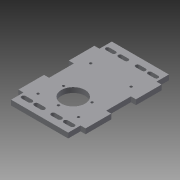
# Autodesk Inventor part: bottom
Saved by Autodesk Inventor 2015 (Build 190159000, 159)
## iProperties
Created: 2017-03-04
Part Number: bottom
Material: Generic
Document SubType Name: Modeling
Designer: Guy
Density: 1 g/cm^3
Appearance: Default
Author: Guy
Autodesk Inventor part; units mm, degrees
ref_plane "YZ Plane" through (0, 0, 0) normal (1, 0, 0) x (0, 1, 0)
ref_plane "XZ Plane" through (0, 0, 0) normal (0, 1, 0) x (-1, 0, 0)
ref_plane "XY Plane" through (0, 0, 0) normal (0, 0, 1) x (1, 0, 0)
sketch "Sketch1" plane through (0, 0, 0) normal (0, 0, 1) x (1, 0, 0)
  line L0 (0, 0) -> (120, 0)
  line L1 (120, 0) -> (120, 80)
  line L2 (120, 80) -> (0, 80)
  line L3 (0, 80) -> (0, 0)
  dimension "d0" = 120
  dimension "d1" = 80
  constraints: 8 end point, 2 parallel, 1 horizontal, 1 perpendicular
  measures "d0" distance of L2.end L1.end
  measures "d1" distance of L0.end L1.end
extrude "Extrusion1" add sketch "Sketch1" along normal blind 6
sketch "Sketch2" plane through (0, 0, 6) normal (0, 0, 1) x (1, 0, 0)
  line L0 (0, 0) -> (120, 0) projected
  line L1 (120, 0) -> (120, 80) projected
  line L2 (120, 80) -> (0, 80) projected
  line L3 (0, 80) -> (0, 0) projected
  line L4 (120, 0) -> (105.25, 0)
  line L5 (105.25, 0) -> (105.25, 6)
  line L6 (105.25, 6) -> (120, 6)
  line L7 (120, 6) -> (120, 0)
  line L8 (0, 0) -> (120, 0) projected
  line L9 (74.75, 0) -> (45.25, 0)
  line L10 (45.25, 0) -> (45.25, 6)
  line L11 (45.25, 6) -> (74.75, 6)
  line L12 (74.75, 6) -> (74.75, 0)
  line L13 (14.75, 0) -> (0, 0)
  line L14 (0, 0) -> (0, 6)
  line L15 (0, 6) -> (14.75, 6)
  line L16 (14.75, 6) -> (14.75, 0)
  line L17 (120, 80) -> (105.25, 80)
  line L18 (105.25, 80) -> (105.25, 74)
  line L19 (105.25, 74) -> (120, 74)
  line L20 (120, 74) -> (120, 80)
  line L21 (120, 80) -> (0, 80) projected
  line L22 (74.75, 80) -> (45.25, 80)
  line L23 (45.25, 80) -> (45.25, 74)
  line L24 (45.25, 74) -> (74.75, 74)
  line L25 (74.75, 74) -> (74.75, 80)
  line L26 (14.75, 80) -> (0, 80)
  line L27 (0, 80) -> (0, 74)
  line L28 (0, 74) -> (14.75, 74)
  line L29 (14.75, 74) -> (14.75, 80)
  line L30 (60, -24.5918) -> (60, 107.6161)
  line L31 (0, 80) -> (0, 0) projected
  dimension "d4" = 6
  dimension "d5" = 6
  dimension "d6" = 14.75
  dimension "d7" = 14.75
  dimension "d8" = 29.5
  dimension "d18" = 60
  dimension "d19" = 14.75
  constraints: 50 end point, 13 parallel, 10 point on line, 6 horizontal, 6 perpendicular, 4 collinear
  measures "d4" distance between parallel lines of L6 L4
  measures "d5" distance between parallel lines of L26 L28
  measures "d6" distance between parallel lines of L5 L1
  measures "d7" distance between parallel lines of L16 L14
  measures "d8" distance between parallel lines of L12 L10
  measures "d18" distance between parallel lines of L3 L30
  measures "d19" distance between parallel lines of L12 L30
extrude "Extrusion2" cut sketch "Sketch2" against normal up to next contours L3 L15 L16 L0 | L10 L11 L30 L0 | L3 L2 L29 L28 | L30 L11 L12 L0 | L5 L6 L1 L0 | L30 L2 L25 L24 | L24 L23 L2 L30 | L19 L18 L2 L1
sketch "Sketch3" plane through (0, 0, 6) normal (0, 0, 1) x (1, 0, 0)
  circle A0 centre (80, 40) radius 4.6
  line L0 (74.75, 0) -> (105.25, 0) projected
  line L1 (120, 6) -> (120, 74) projected
  point P0 (0, 0)
  dimension "d13" = 9.2
  dimension "d14" = 40
  dimension "d15" = 40
  constraints: 1 centre point
  measures "d13" diameter of A0
  measures "d14" distance from line of A0.centre L0
  measures "d15" distance from line of L1 A0.centre
extrude "Extrusion3" cut sketch "Sketch3" against normal up to next
sketch "Sketch4" plane through (0, 0, 6) normal (0, 0, 1) x (1, 0, 0)
  circle A0 centre (80, 40) radius 4.6 projected
  line L0 (74.75, 6) -> (74.75, 0) projected
  line L1 (74.75, 0) -> (105.25, 0) projected
  line L2 (105.25, 0) -> (105.25, 6) projected
  line L3 (105.25, 6) -> (120, 6) projected
  line L4 (120, 6) -> (120, 74) projected
  line L5 (120, 74) -> (105.25, 74) projected
  line L6 (105.25, 74) -> (105.25, 80) projected
  line L7 (105.25, 80) -> (74.75, 80) projected
  line L8 (74.75, 80) -> (74.75, 74) projected
  line L9 (74.75, 74) -> (45.25, 74) projected
  line L10 (45.25, 74) -> (45.25, 80) projected
  line L11 (45.25, 80) -> (14.75, 80) projected
  line L12 (14.75, 80) -> (14.75, 74) projected
  line L13 (14.75, 74) -> (0, 74) projected
  line L14 (0, 74) -> (0, 6) projected
  line L15 (0, 6) -> (14.75, 6) projected
  line L16 (14.75, 6) -> (14.75, 0) projected
  line L17 (14.75, 0) -> (45.25, 0) projected
  line L18 (45.25, 0) -> (45.25, 6) projected
  line L19 (45.25, 6) -> (74.75, 6) projected
  circle A1 centre (80, 40) radius 14.125
  circle A2 centre (97.5, 40) radius 1.5
  circle A3 centre (74.5, 57) radius 1.5
  circle A4 centre (74.5, 23) radius 1.5
  circle A5 centre (35.064, 64.1) radius 1.5
  circle A6 centre (35.064, 15.9) radius 1.5
  line L20 (80, 40) -> (97.5, 40) construction
  circle A7 centre (10, 66.125) radius 2.3
  circle A8 centre (10, 51.125) radius 2.3
  circle A9 centre (10, 13.875) radius 2.3
  circle A10 centre (10, 28.875) radius 2.3
  circle A11 centre (110, 66.125) radius 2.5
  circle A12 centre (110, 51.125) radius 2.5
  circle A13 centre (110, 13.875) radius 2.5
  circle A14 centre (110, 28.875) radius 2.5
  line L21 (10, 66.125) -> (110, 66.125) construction
  line L22 (110, 66.125) -> (110, 13.875) construction
  line L23 (110, 13.875) -> (10, 13.875) construction
  line L24 (10, 13.875) -> (10, 66.125) construction
  circle A15 centre (10, 61.125) radius 2.3
  circle A16 centre (10, 54.125) radius 2.3
  circle A17 centre (10, 69.125) radius 2.3
  circle A18 centre (10, 46.525) radius 2.3
  circle A19 centre (10, 33.475) radius 2.3
  circle A20 centre (10, 25.875) radius 2.3
  circle A21 centre (10, 18.475) radius 2.3
  circle A22 centre (10, 10.875) radius 2.3
  circle A23 centre (110, 69.125) radius 2.5
  circle A24 centre (110, 61.125) radius 2.5
  circle A25 centre (110, 54.125) radius 2.5
  circle A26 centre (110, 46.125) radius 2.5
  circle A27 centre (110, 33.875) radius 2.5
  circle A28 centre (110, 25.875) radius 2.5
  circle A29 centre (110, 18.875) radius 2.5
  circle A30 centre (110, 10.875) radius 2.5
  line L25 (7.7, 69.125) -> (7.7, 61.125)
  line L26 (12.3, 61.125) -> (12.3, 69.125)
  line L27 (7.7, 54.125) -> (7.7, 46.525)
  line L28 (12.3, 46.525) -> (12.3, 54.125)
  line L29 (7.7, 10.875) -> (7.7, 18.475)
  line L30 (7.7, 25.875) -> (7.7, 33.475)
  line L31 (12.3, 33.475) -> (12.3, 25.875)
  line L32 (12.3, 18.475) -> (12.3, 10.875)
  line L33 (112.5, 61.125) -> (112.5, 69.125)
  line L34 (107.5, 69.125) -> (107.5, 61.125)
  line L35 (107.5, 54.125) -> (107.5, 46.125)
  line L36 (112.5, 46.125) -> (112.5, 54.125)
  line L37 (107.5, 33.875) -> (107.5, 25.875)
  line L38 (107.5, 18.875) -> (107.5, 10.875)
  line L39 (112.5, 10.875) -> (112.5, 18.875)
  line L40 (112.5, 25.875) -> (112.5, 33.875)
  point P0 (0, 0)
  dimension "d20" = 28.25
  dimension "d21" = 3
  dimension "d22" = 3
  dimension "d23" = 3
  dimension "d24" = 3
  dimension "d25" = 3
  dimension "d26" = 17.5
  dimension "d27" = 5.5
  dimension "d28" = 5.5
  dimension "d29" = 34
  dimension "d30" = 17
  dimension "d31" = 48.2
  dimension "d32" = 24.1
  dimension "d33" = 44.936
  dimension "d34" = 44.936
  dimension "d37" = 10
  dimension "d38" = 10
  dimension "d39" = 4.6
  dimension "d40" = 4.6
  dimension "d41" = 4.6
  dimension "d42" = 4.6
  dimension "d43" = 5
  dimension "d44" = 5
  dimension "d45" = 5
  dimension "d46" = 5
  dimension "d47" = 13.875
  dimension "d48" = 13.875
  dimension "d49" = 15
  dimension "d50" = 15
  dimension "d51" = 15
  dimension "d52" = 15
  dimension "d53" = 4.6
  dimension "d54" = 4.6
  dimension "d56" = 3
  dimension "d57" = 5
  dimension "d58" = 4.6
  dimension "d59" = 3
  dimension "d60" = 4.6
  dimension "d61" = 4.6
  dimension "d62" = 4.6
  dimension "d63" = 4.6
  dimension "d64" = 4.6
  dimension "d65" = 3
  dimension "d66" = 3
  dimension "d67" = 5
  dimension "d68" = 5
  dimension "d69" = 5
  dimension "d70" = 5
  dimension "d71" = 5
  dimension "d72" = 5
  dimension "d73" = 5
  dimension "d74" = 5
  dimension "d75" = 3
  dimension "d76" = 3
  dimension "d77" = 3
  dimension "d78" = 3
  constraints: 38 end point, 34 tangent, 32 point on circle, 30 centre point, 4 vertical, 3 coincident, 3 horizontal, 1 parallel, 1 point on line, 26 other
  measures "d20" diameter of A1
  measures "d21" diameter of A5
  measures "d22" diameter of A6
  measures "d23" diameter of A3
  measures "d24" diameter of A4
  measures "d25" diameter of A2
  measures "d26" distance of A0.centre L20.end
  measures "d27" horizontal distance of A0.centre A3.centre
  measures "d28" horizontal distance of A0.centre A4.centre
  measures "d29" distance of A3.centre A4.centre
  measures "d30" vertical distance of A3.centre L20.start
  measures "d31" distance of A6.centre A5.centre
  measures "d32" vertical distance of A0.centre A5.centre
  measures "d33" horizontal distance of A0.centre A5.centre
  measures "d34" horizontal distance of L20.start A6.centre
  measures "d39" diameter of A7
  measures "d40" diameter of A8
  measures "d41" diameter of A9
  measures "d42" diameter of A10
  measures "d43" diameter of A13
  measures "d44" diameter of A14
  measures "d45" diameter of A12
  measures "d46" diameter of A11
  measures "d47" distance between parallel lines of L11 L21
  measures "d48" distance between parallel lines of L23 L17
  measures "d49" distance of A8.centre L21.start
  measures "d50" distance of A9.centre A10.centre
  measures "d51" distance of A12.centre A11.centre
  measures "d52" distance from line of L23 A14.centre
  measures "d53" diameter of A15
  measures "d54" diameter of A16
  measures "d56" distance of A16.centre A8.centre
  measures "d57" distance of A15.centre L21.start
  measures "d58" diameter of A17
  measures "d59" distance of L21.start A17.centre
  measures "d60" diameter of A18
  measures "d61" diameter of A19
  measures "d62" diameter of A20
  measures "d63" diameter of A21
  measures "d64" diameter of A22
  measures "d65" distance of A9.centre A22.centre
  measures "d66" distance of A10.centre A20.centre
  measures "d67" diameter of A23
  measures "d68" diameter of A24
  measures "d69" diameter of A25
  measures "d70" diameter of A26
  measures "d71" diameter of A27
  measures "d72" diameter of A28
  measures "d73" diameter of A29
  measures "d74" diameter of A30
  measures "d75" distance of L23.start A30.centre
  measures "d76" distance of A11.centre A23.centre
  measures "d77" distance of A12.centre A25.centre
  measures "d78" distance of A14.centre A28.centre
extrude "Extrusion4" cut sketch "Sketch4" against normal blind 10 contours A1 | A2 | A3 | A4 | A5 | A6
extrude "Extrusion5" cut sketch "Sketch4" against normal blind 10 contours A7 A17 | L26 A15 L25 A7 | A7 A17 L26 | A17 A7 | A7 A17 | L25 A17 A7 | A15 | A8 A16 | L28 A18 A8 | A8 A16 L28 | A16 A8 | A8 A16 | A18 L27 A8 | A18 | A8 L27 A16 | A9 A22 | L32 A22 A9 | A9 A21 L32 | A9 L29 A21 | A21 | A22 A9 | A9 A22 | A9 A22 L29 | A10 A20 | L31 A20 A10 | A10 A19 L31 | A10 L30 A19 | A19 | A20 A10 | A10 A20 | A10 A20 L30 | A11 A23 | L33 A24 A11 | A11 A23 L33 | A23 A11 | A11 A23 | A24 L34 A11 | A24 | A11 L34 A23 | A12 A25 | L36 A26 A12 | A12 A25 L36 | A25 A12 | A12 A25 | A26 L35 A12 | A26 | A12 L35 A25 | A13 A30 | L39 A30 A13 | A13 A29 L39 | A13 L38 A29 | A29 | A30 A13 | A13 A30 | A13 A30 L38 | A14 A28 | L40 A28 A14 | A14 A27 L40 | A14 L37 A27 | A27 | A28 A14 | A14 A28 | A14 A28 L37
sketch "Sketch6" plane through (0, 0, 6) normal (0, 0, 1) x (1, 0, 0)
  line L0 (107.5, 25.875) -> (107.5, 33.875) projected
  arc A0 (112.5, 33.875) -> (107.5, 33.875) centre (110, 33.875) ccw projected
  line L1 (112.5, 33.875) -> (112.5, 25.875) projected
  arc A1 (107.5, 25.875) -> (112.5, 25.875) centre (110, 25.875) ccw projected
  line L2 (7.7, 25.875) -> (7.7, 33.475) projected
  arc A2 (12.3, 33.475) -> (7.7, 33.475) centre (10, 33.475) ccw projected
  line L3 (12.3, 33.475) -> (12.3, 25.875) projected
  arc A3 (7.7, 25.875) -> (12.3, 25.875) centre (10, 25.875) ccw projected
  line L4 (12.3, 54.125) -> (12.3, 46.525) projected
  arc A4 (7.7, 46.525) -> (12.3, 46.525) centre (10, 46.525) ccw projected
  line L5 (7.7, 46.525) -> (7.7, 54.125) projected
  arc A5 (12.3, 54.125) -> (7.7, 54.125) centre (10, 54.125) ccw projected
  line L6 (7.7, 10.875) -> (7.7, 18.475) projected
  arc A6 (12.3, 18.475) -> (7.7, 18.475) centre (10, 18.475) ccw projected
  line L7 (12.3, 18.475) -> (12.3, 10.875) projected
  arc A7 (7.7, 10.875) -> (12.3, 10.875) centre (10, 10.875) ccw projected
  line L8 (107.5, 61.125) -> (107.5, 69.125) projected
  arc A8 (112.5, 69.125) -> (107.5, 69.125) centre (110, 69.125) ccw projected
  line L9 (112.5, 69.125) -> (112.5, 61.125) projected
  arc A9 (107.5, 61.125) -> (112.5, 61.125) centre (110, 61.125) ccw projected
  line L10 (112.5, 18.875) -> (112.5, 10.875) projected
  arc A10 (107.5, 10.875) -> (112.5, 10.875) centre (110, 10.875) ccw projected
  line L11 (107.5, 10.875) -> (107.5, 18.875) projected
  arc A11 (112.5, 18.875) -> (107.5, 18.875) centre (110, 18.875) ccw projected
  line L12 (7.7, 61.125) -> (7.7, 69.125) projected
  arc A12 (12.3, 69.125) -> (7.7, 69.125) centre (10, 69.125) ccw projected
  line L13 (12.3, 69.125) -> (12.3, 61.125) projected
  arc A13 (7.7, 61.125) -> (12.3, 61.125) centre (10, 61.125) ccw projected
  line L14 (112.5, 54.125) -> (112.5, 46.125) projected
  arc A14 (107.5, 46.125) -> (112.5, 46.125) centre (110, 46.125) ccw projected
  line L15 (107.5, 46.125) -> (107.5, 54.125) projected
  arc A15 (112.5, 54.125) -> (107.5, 54.125) centre (110, 54.125) ccw projected
  circle A16 centre (80, 40) radius 14.125 projected
  circle A17 centre (35.064, 64.1) radius 1.5 projected
  circle A18 centre (74.5, 57) radius 1.5 projected
  circle A19 centre (97.5, 40) radius 1.5 projected
  circle A20 centre (74.5, 23) radius 1.5 projected
  circle A21 centre (35.064, 15.9) radius 1.5 projected
  line L16 (74.75, 6) -> (74.75, 0) projected
  line L17 (74.75, 0) -> (105.25, 0) projected
  line L18 (105.25, 0) -> (105.25, 6) projected
  line L19 (105.25, 6) -> (120, 6) projected
  line L20 (120, 6) -> (120, 74) projected
  line L21 (120, 74) -> (105.25, 74) projected
  line L22 (105.25, 74) -> (105.25, 80) projected
  line L23 (105.25, 80) -> (74.75, 80) projected
  line L24 (74.75, 80) -> (74.75, 74) projected
  line L25 (74.75, 74) -> (45.25, 74) projected
  line L26 (45.25, 74) -> (45.25, 80) projected
  line L27 (45.25, 80) -> (14.75, 80) projected
  line L28 (14.75, 80) -> (14.75, 74) projected
  line L29 (14.75, 74) -> (0, 74) projected
  line L30 (0, 74) -> (0, 6) projected
  line L31 (0, 6) -> (14.75, 6) projected
  line L32 (14.75, 6) -> (14.75, 0) projected
  line L33 (14.75, 0) -> (45.25, 0) projected
  line L34 (45.25, 0) -> (45.25, 6) projected
  line L35 (45.25, 6) -> (74.75, 6) projected
  circle A22 centre (97.765, 15.9) radius 1.5
  circle A23 centre (97.765, 64.1) radius 1.5
  point P0 (0, 0)
  dimension "d94" = 62.701
  dimension "d95" = 15.9
  dimension "d96" = 15.9
  dimension "d97" = 3
  dimension "d98" = 62.701
  dimension "d99" = 15.9
  dimension "d100" = 3
  constraints: 2 centre point
  measures "d94" distance of A22.centre A21.centre
  measures "d95" distance from line of L33 A21.centre
  measures "d96" distance from line of L17 A22.centre
  measures "d97" diameter of A22
  measures "d98" distance of A17.centre A23.centre
  measures "d99" distance from line of L23 A23.centre
  measures "d100" diameter of A23
extrude "Extrusion7" cut sketch "Sketch6" against normal blind 10 contours A22 | A23
equation "\"d22\" = d21"
equation "\"d23\" = d21"
equation "\"d24\" = d21"
equation "\"d25\" = d21"
equation "\"d30\" = 0.5 * d29"
equation "\"d32\" = 0.5 * d31"
equation "\"d34\" = d33"
equation "\"d39\" = d64"
equation "\"d40\" = d64"
equation "\"d41\" = d64"
equation "\"d42\" = d64"
equation "\"d43\" = d74"
equation "\"d44\" = d74"
equation "\"d45\" = d74"
equation "\"d46\" = d74"
equation "\"d48\" = d47"
equation "\"d53\" = d64"
equation "\"d54\" = d64"
equation "\"d58\" = d64"
equation "\"d60\" = d64"
equation "\"d61\" = d64"
equation "\"d62\" = d64"
equation "\"d63\" = d64"
equation "\"d67\" = d74"
equation "\"d68\" = d74"
equation "\"d69\" = d74"
equation "\"d70\" = d74"
equation "\"d71\" = d74"
equation "\"d72\" = d74"
equation "\"d73\" = d74"
equation "\"d96\" = d95"
equation "\"d98\" = d94"
equation "\"d99\" = d96"
body "Solid1"
